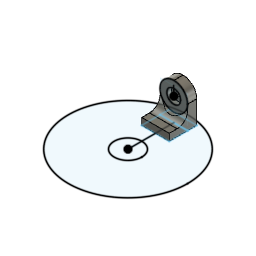
Wing Hinge v2 (Autodesk Fusion 360 design; units mm, degrees)
Autodesk Fusion 360 part; units mm, degrees
sketch "Sketch1" plane through (0, 0, 0) normal (0, 1, 0) x (1, 0, 0)
  circle A0 centre (0, 0) radius 13
  circle A1 centre (0, 0) radius 3
  line L0 (0, 0) -> (0, 10)
  line L1 (0, 10) -> (3, 10)
  line L2 (3, 10) -> (3, 12)
  line L3 (3, 12) -> (-3, 12)
  line L4 (-3, 12) -> (-3, 10)
  line L5 (-3, 10) -> (3, 10)
  line L6 (-3, 10) -> (3, 10)
  line L7 (3, 10) -> (3, 6)
  line L8 (3, 6) -> (-3, 6)
  line L9 (-3, 6) -> (-3, 10)
  dimension "d1" = 26
  dimension "d2" = 6
  constraint coincident A0.centre A1.centre
  constraint concentric A0 A1
  constraint vertical L0
  constraint perpendicular L0 L1
  constraint perpendicular L1 L2
  constraint perpendicular L2 L3
  constraint perpendicular L3 L4
  constraint perpendicular L4 L5
  constraint horizontal L6
  constraint vertical L7
  constraint horizontal L8
  constraint vertical L9
  measures "d1" diameter of A0
  measures "d2" diameter of A1
extrude "Extrude1" add sketch "Sketch1" along normal blind 1 contours L0 L5 L6 L8 L9 | L0 L1 L5 L6 L7 L8
extrude "Extrude2" add sketch "Sketch1" along normal blind 6 contours L1 L2 L3 L4 L5 L6
extrude "Extrude3" add 1 faces at (-1, 6, -11.3333) along direction (0, 1, 0) blind 1
sketch "Sketch2" plane through (0, 0, -10) normal (0, 0, 1) x (1, 0, 0)
  line L0 (-3, 1) -> (3, 1)
  line L1 (3, 1) -> (3, 7)
  line L2 (3, 7) -> (-3, 7)
  line L3 (-3, 7) -> (-3, 1)
  line L4 (0, 7) -> (0, 5)
  circle A0 centre (0, 5) radius 0.5
  circle A1 centre (0, 5) radius 3
  circle A2 centre (0, 5) radius 1.5
  dimension "d9" = 2
  dimension "d10" = 1
  dimension "d23" = 3
  constraint midpoint L2 L4.start
  constraint perpendicular L2 L4
  constraint coincident L4.end A0.centre
  constraint concentric A0 A1
  constraint tangent L1 A1
  constraint concentric A0 A2
  measures "d9" distance of L4.start L4.end
  measures "d10" diameter of A0
  measures "d23" diameter of A2
extrude "Extrude4" cut sketch "Sketch2" against normal blind 5.8 contours A0
extrude "Extrude5" add 1 faces at (1, 1, -7.3333) along direction (0, 1, 0) blind 1
extrude "Extrude6" cut 1 faces at (1, 2, -7.3333) along direction (0, -1, 0) blind 0.5
extrude "Extrude7" cut sketch "Sketch2" against normal blind 1 contours L2 A1 | A2 picked at (-0.9591, 6.7853)
fillet "Fillet1" radius 2.3 1 edges at (0, 1.5, -10)
extrude "Extrude8" add 1 faces at (-0.0125, 6.4995, -11) along direction (0, 0, 1) blind 1
extrude "Extrude9" add 1 faces at (-1, 7, -11.3333) along direction (0, 1, 0) blind 1
extrude "Extrude10" cut sketch "Sketch2" against normal blind 1 contours A2
fillet "Fillet2" radius 3 2 edges at (-3, 8, -11) (3, 8, -11)
